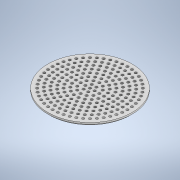
# Autodesk Inventor part: Filter Plate
Saved by Autodesk Inventor 2022 (Build 260153000, 153)
## iProperties
Created: 2022-05-11
Part Number: Filter Plate
Material: Generic
Document SubType Name: Modeling
Designer: efred
Density: 1 g/cm^3
Appearance: Default
Author: efred
Autodesk Inventor part; units mm, degrees
ref_plane "YZ Plane" through (0, 0, 0) normal (1, 0, 0) x (0, 1, 0)
ref_plane "XZ Plane" through (0, 0, 0) normal (0, 1, 0) x (-1, 0, 0)
ref_plane "XY Plane" through (0, 0, 0) normal (0, 0, 1) x (1, 0, 0)
sketch "Sketch1" plane through (0, 0, 0) normal (0, 1, 0) x (-1, 0, 0)
  circle A0 centre (0, 0) radius 13.5
  circle A1 centre (0, 0) radius 0.4
  line L0 (0, 0) -> (13.5, 0) construction
  circle A2 centre (1.5, 0) radius 0.4
  circle A3 centre (3, 0) radius 0.4
  circle A4 centre (4.5, 0) radius 0.4
  circle A5 centre (6, 0) radius 0.4
  circle A6 centre (7.5, 0) radius 0.4
  circle A7 centre (9, 0) radius 0.4
  circle A8 centre (10.5, 0) radius 0.4
  circle A9 centre (12, 0) radius 0.4
  circle A10 centre (0.75, 1.299) radius 0.4
  circle A11 centre (-0.75, 1.299) radius 0.4
  circle A12 centre (-1.5, 0) radius 0.4
  circle A13 centre (-0.75, -1.299) radius 0.4
  circle A14 centre (0.75, -1.299) radius 0.4
  circle A15 centre (2.5981, 1.5) radius 0.4
  circle A16 centre (1.5, 2.5981) radius 0.4
  circle A17 centre (0, 3) radius 0.4
  circle A18 centre (-1.5, 2.5981) radius 0.4
  circle A19 centre (-2.5981, 1.5) radius 0.4
  circle A20 centre (-3, 0) radius 0.4
  circle A21 centre (-2.5981, -1.5) radius 0.4
  circle A22 centre (-1.5, -2.5981) radius 0.4
  circle A23 centre (0, -3) radius 0.4
  circle A24 centre (1.5, -2.5981) radius 0.4
  circle A25 centre (2.5981, -1.5) radius 0.4
  circle A26 centre (4.2286, 1.5391) radius 0.4
  circle A27 centre (3.4472, 2.8925) radius 0.4
  circle A28 centre (2.25, 3.8971) radius 0.4
  circle A29 centre (0.7814, 4.4316) radius 0.4
  circle A30 centre (-0.7814, 4.4316) radius 0.4
  circle A31 centre (-2.25, 3.8971) radius 0.4
  circle A32 centre (-3.4472, 2.8925) radius 0.4
  circle A33 centre (-4.2286, 1.5391) radius 0.4
  circle A34 centre (-4.5, 0) radius 0.4
  circle A35 centre (-4.2286, -1.5391) radius 0.4
  circle A36 centre (-3.4472, -2.8925) radius 0.4
  circle A37 centre (-2.25, -3.8971) radius 0.4
  circle A38 centre (-0.7814, -4.4316) radius 0.4
  circle A39 centre (0.7814, -4.4316) radius 0.4
  circle A40 centre (2.25, -3.8971) radius 0.4
  circle A41 centre (3.4472, -2.8925) radius 0.4
  circle A42 centre (4.2286, -1.5391) radius 0.4
  circle A43 centre (5.7956, 1.5529) radius 0.4
  circle A44 centre (5.1962, 3) radius 0.4
  circle A45 centre (4.2426, 4.2426) radius 0.4
  circle A46 centre (3, 5.1962) radius 0.4
  circle A47 centre (1.5529, 5.7956) radius 0.4
  circle A48 centre (0, 6) radius 0.4
  circle A49 centre (-1.5529, 5.7956) radius 0.4
  circle A50 centre (-3, 5.1962) radius 0.4
  circle A51 centre (-4.2426, 4.2426) radius 0.4
  circle A52 centre (-5.1962, 3) radius 0.4
  circle A53 centre (-5.7956, 1.5529) radius 0.4
  circle A54 centre (-6, 0) radius 0.4
  circle A55 centre (-5.7956, -1.5529) radius 0.4
  circle A56 centre (-5.1962, -3) radius 0.4
  circle A57 centre (-4.2426, -4.2426) radius 0.4
  circle A58 centre (-3, -5.1962) radius 0.4
  circle A59 centre (-1.5529, -5.7956) radius 0.4
  circle A60 centre (0, -6) radius 0.4
  circle A61 centre (1.5529, -5.7956) radius 0.4
  circle A62 centre (3, -5.1962) radius 0.4
  circle A63 centre (4.2426, -4.2426) radius 0.4
  circle A64 centre (5.1962, -3) radius 0.4
  circle A65 centre (5.7956, -1.5529) radius 0.4
  circle A66 centre (7.3361, 1.5593) radius 0.4
  circle A67 centre (6.8516, 3.0505) radius 0.4
  circle A68 centre (6.0676, 4.4084) radius 0.4
  circle A69 centre (5.0185, 5.5736) radius 0.4
  circle A70 centre (3.75, 6.4952) radius 0.4
  circle A71 centre (2.3176, 7.1329) radius 0.4
  circle A72 centre (0.784, 7.4589) radius 0.4
  circle A73 centre (-0.784, 7.4589) radius 0.4
  circle A74 centre (-2.3176, 7.1329) radius 0.4
  circle A75 centre (-3.75, 6.4952) radius 0.4
  circle A76 centre (-5.0185, 5.5736) radius 0.4
  circle A77 centre (-6.0676, 4.4084) radius 0.4
  circle A78 centre (-6.8516, 3.0505) radius 0.4
  circle A79 centre (-7.3361, 1.5593) radius 0.4
  circle A80 centre (-7.5, 0) radius 0.4
  circle A81 centre (-7.3361, -1.5593) radius 0.4
  circle A82 centre (-6.8516, -3.0505) radius 0.4
  circle A83 centre (-6.0676, -4.4084) radius 0.4
  circle A84 centre (-5.0185, -5.5736) radius 0.4
  circle A85 centre (-3.75, -6.4952) radius 0.4
  circle A86 centre (-2.3176, -7.1329) radius 0.4
  circle A87 centre (-0.784, -7.4589) radius 0.4
  circle A88 centre (0.784, -7.4589) radius 0.4
  circle A89 centre (2.3176, -7.1329) radius 0.4
  circle A90 centre (3.75, -6.4952) radius 0.4
  circle A91 centre (5.0185, -5.5736) radius 0.4
  circle A92 centre (6.0676, -4.4084) radius 0.4
  circle A93 centre (6.8516, -3.0505) radius 0.4
  circle A94 centre (7.3361, -1.5593) radius 0.4
  circle A95 centre (8.8633, 1.5628) radius 0.4
  circle A96 centre (8.4572, 3.0782) radius 0.4
  circle A97 centre (7.7942, 4.5) radius 0.4
  circle A98 centre (6.8944, 5.7851) radius 0.4
  circle A99 centre (5.7851, 6.8944) radius 0.4
  circle A100 centre (4.5, 7.7942) radius 0.4
  circle A101 centre (3.0782, 8.4572) radius 0.4
  circle A102 centre (1.5628, 8.8633) radius 0.4
  circle A103 centre (0, 9) radius 0.4
  circle A104 centre (-1.5628, 8.8633) radius 0.4
  circle A105 centre (-3.0782, 8.4572) radius 0.4
  circle A106 centre (-4.5, 7.7942) radius 0.4
  circle A107 centre (-5.7851, 6.8944) radius 0.4
  circle A108 centre (-6.8944, 5.7851) radius 0.4
  circle A109 centre (-7.7942, 4.5) radius 0.4
  circle A110 centre (-8.4572, 3.0782) radius 0.4
  circle A111 centre (-8.8633, 1.5628) radius 0.4
  circle A112 centre (-9, 0) radius 0.4
  circle A113 centre (-8.8633, -1.5628) radius 0.4
  circle A114 centre (-8.4572, -3.0782) radius 0.4
  circle A115 centre (-7.7942, -4.5) radius 0.4
  circle A116 centre (-6.8944, -5.7851) radius 0.4
  circle A117 centre (-5.7851, -6.8944) radius 0.4
  circle A118 centre (-4.5, -7.7942) radius 0.4
  circle A119 centre (-3.0782, -8.4572) radius 0.4
  circle A120 centre (-1.5628, -8.8633) radius 0.4
  circle A121 centre (0, -9) radius 0.4
  circle A122 centre (1.5628, -8.8633) radius 0.4
  circle A123 centre (3.0782, -8.4572) radius 0.4
  circle A124 centre (4.5, -7.7942) radius 0.4
  circle A125 centre (5.7851, -6.8944) radius 0.4
  circle A126 centre (6.8944, -5.7851) radius 0.4
  circle A127 centre (7.7942, -4.5) radius 0.4
  circle A128 centre (8.4572, -3.0782) radius 0.4
  circle A129 centre (8.8633, -1.5628) radius 0.4
  circle A130 centre (10.3827, 1.5649) radius 0.4
  circle A131 centre (10.0335, 3.0949) radius 0.4
  circle A132 centre (9.4602, 4.5558) radius 0.4
  circle A133 centre (8.6755, 5.9149) radius 0.4
  circle A134 centre (7.697, 7.1418) radius 0.4
  circle A135 centre (6.5466, 8.2092) radius 0.4
  circle A136 centre (5.25, 9.0933) radius 0.4
  circle A137 centre (3.8361, 9.7742) radius 0.4
  circle A138 centre (2.3365, 10.2367) radius 0.4
  circle A139 centre (0.7847, 10.4706) radius 0.4
  circle A140 centre (-0.7847, 10.4706) radius 0.4
  circle A141 centre (-2.3365, 10.2367) radius 0.4
  circle A142 centre (-3.8361, 9.7742) radius 0.4
  circle A143 centre (-5.25, 9.0933) radius 0.4
  circle A144 centre (-6.5466, 8.2092) radius 0.4
  circle A145 centre (-7.697, 7.1418) radius 0.4
  circle A146 centre (-8.6755, 5.9149) radius 0.4
  circle A147 centre (-9.4602, 4.5558) radius 0.4
  circle A148 centre (-10.0335, 3.0949) radius 0.4
  circle A149 centre (-10.3827, 1.5649) radius 0.4
  circle A150 centre (-10.5, 0) radius 0.4
  circle A151 centre (-10.3827, -1.5649) radius 0.4
  circle A152 centre (-10.0335, -3.0949) radius 0.4
  circle A153 centre (-9.4602, -4.5558) radius 0.4
  circle A154 centre (-8.6755, -5.9149) radius 0.4
  circle A155 centre (-7.697, -7.1418) radius 0.4
  circle A156 centre (-6.5466, -8.2092) radius 0.4
  circle A157 centre (-5.25, -9.0933) radius 0.4
  circle A158 centre (-3.8361, -9.7742) radius 0.4
  circle A159 centre (-2.3365, -10.2367) radius 0.4
  circle A160 centre (-0.7847, -10.4706) radius 0.4
  circle A161 centre (0.7847, -10.4706) radius 0.4
  circle A162 centre (2.3365, -10.2367) radius 0.4
  circle A163 centre (3.8361, -9.7742) radius 0.4
  circle A164 centre (5.25, -9.0933) radius 0.4
  circle A165 centre (6.5466, -8.2092) radius 0.4
  circle A166 centre (7.697, -7.1418) radius 0.4
  circle A167 centre (8.6755, -5.9149) radius 0.4
  circle A168 centre (9.4602, -4.5558) radius 0.4
  circle A169 centre (10.0335, -3.0949) radius 0.4
  circle A170 centre (10.3827, -1.5649) radius 0.4
  circle A171 centre (11.8973, 1.5663) radius 0.4
  circle A172 centre (11.5911, 3.1058) radius 0.4
  circle A173 centre (11.0866, 4.5922) radius 0.4
  circle A174 centre (10.3923, 6) radius 0.4
  circle A175 centre (9.5202, 7.3051) radius 0.4
  circle A176 centre (8.4853, 8.4853) radius 0.4
  circle A177 centre (7.3051, 9.5202) radius 0.4
  circle A178 centre (6, 10.3923) radius 0.4
  circle A179 centre (4.5922, 11.0866) radius 0.4
  circle A180 centre (3.1058, 11.5911) radius 0.4
  circle A181 centre (1.5663, 11.8973) radius 0.4
  circle A182 centre (0, 12) radius 0.4
  circle A183 centre (-1.5663, 11.8973) radius 0.4
  circle A184 centre (-3.1058, 11.5911) radius 0.4
  circle A185 centre (-4.5922, 11.0866) radius 0.4
  circle A186 centre (-6, 10.3923) radius 0.4
  circle A187 centre (-7.3051, 9.5202) radius 0.4
  circle A188 centre (-8.4853, 8.4853) radius 0.4
  circle A189 centre (-9.5202, 7.3051) radius 0.4
  circle A190 centre (-10.3923, 6) radius 0.4
  circle A191 centre (-11.0866, 4.5922) radius 0.4
  circle A192 centre (-11.5911, 3.1058) radius 0.4
  circle A193 centre (-11.8973, 1.5663) radius 0.4
  circle A194 centre (-12, 0) radius 0.4
  circle A195 centre (-11.8973, -1.5663) radius 0.4
  circle A196 centre (-11.5911, -3.1058) radius 0.4
  circle A197 centre (-11.0866, -4.5922) radius 0.4
  circle A198 centre (-10.3923, -6) radius 0.4
  circle A199 centre (-9.5202, -7.3051) radius 0.4
  circle A200 centre (-8.4853, -8.4853) radius 0.4
  circle A201 centre (-7.3051, -9.5202) radius 0.4
  circle A202 centre (-6, -10.3923) radius 0.4
  circle A203 centre (-4.5922, -11.0866) radius 0.4
  circle A204 centre (-3.1058, -11.5911) radius 0.4
  circle A205 centre (-1.5663, -11.8973) radius 0.4
  circle A206 centre (0, -12) radius 0.4
  circle A207 centre (1.5663, -11.8973) radius 0.4
  circle A208 centre (3.1058, -11.5911) radius 0.4
  circle A209 centre (4.5922, -11.0866) radius 0.4
  circle A210 centre (6, -10.3923) radius 0.4
  circle A211 centre (7.3051, -9.5202) radius 0.4
  circle A212 centre (8.4853, -8.4853) radius 0.4
  circle A213 centre (9.5202, -7.3051) radius 0.4
  circle A214 centre (10.3923, -6) radius 0.4
  circle A215 centre (11.0866, -4.5922) radius 0.4
  circle A216 centre (11.5911, -3.1058) radius 0.4
  circle A217 centre (11.8973, -1.5663) radius 0.4
  dimension "d0" = 27
  dimension "d1" = 0.8
  dimension "d4" = 1.5
  dimension "d11" = 360
  dimension "d15" = 360
  dimension "d19" = 360
  dimension "d23" = 360
  dimension "d27" = 360
  dimension "d31" = 360
  dimension "d35" = 360
  dimension "d39" = 360
  constraints: 217 centre point, 2 coincident, 2 end point, 2 horizontal, 1 horizontal alignment, 458 other
  measures "d1" diameter of A1
  measures "d4" distance of L0.start A2.centre
extrude "Extrusion1" add sketch "Sketch1" along normal blind 1
chamfer "Chamfer1" distance 0.5 angle 45 1 edges at (13.5, 0, 0)
body "Solid1"
